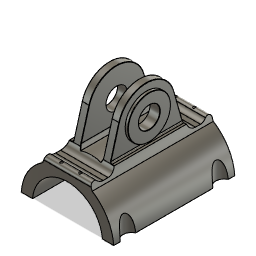
0.885.7050 - Demi-bride à chape pour tube 49 - IGTE 21485_232872 (Autodesk Fusion 360 design; units mm, degrees)
Autodesk Fusion 360 part; units mm, degrees
sketch "Sketch1" plane through (0, 0, 0) normal (0, 0, 1) x (1, 0, 0)
  line L0 (0, 0) -> (50, 0) construction
  line L1 (0, 0) -> (0, 2) construction
  line L2 (0, 0) -> (-50, 0) construction
  line L3 (0, 2) -> (50, 2) construction
  line L4 (0, 2) -> (-50, 2) construction
  arc A0 (24.5186, 2) -> (-24.5186, 2) centre (0, 0) ccw
  arc A1 (32.4384, 2) -> (-32.4384, 2) centre (0, 0) ccw
  line L5 (24.5186, 2) -> (32.4384, 2)
  line L6 (-32.4384, 2) -> (-24.5186, 2)
  line L7 (0, 50) -> (50, 50) construction
  line L8 (0, 50) -> (-50, 50) construction
  line L9 (0, 65) -> (50, 65) construction
  line L10 (0, 65) -> (-50, 65) construction
  line L11 (0, 70) -> (-50, 70) construction
  line L12 (0, 70) -> (50, 70) construction
  line L13 (0, 2) -> (0, 70) construction
  line L14 (8, 0) -> (8, 2) construction
  line L15 (8, 2) -> (8, 70) construction
  line L16 (-8, 0) -> (-8, 2) construction
  line L17 (-8, 2) -> (-8, 70) construction
  line L18 (13, 0) -> (13, 2) construction
  line L19 (-13, 0) -> (-13, 2) construction
  line L20 (-13, 2) -> (-13, 70) construction
  line L21 (15, 0) -> (15, 2) construction
  line L22 (15, 40.9995) -> (15, 65)
  line L23 (-15, 0) -> (-15, 2) construction
  line L24 (-15, 2) -> (-15, 65) construction
  arc A2 (28.931, 2) -> (-28.931, 2) centre (0, 0) ccw construction
  arc A3 (28.53, 2) -> (22.93, 17.0931) centre (0, 0) ccw
  line L25 (8, 70) -> (13, 70)
  line L26 (8, 70) -> (8, 35)
  line L27 (0, 29) -> (2, 29)
  arc A4 (2, 29) -> (8, 35) centre (2, 35) ccw
  arc A5 (-8, 35) -> (-2, 29) centre (-2, 35) ccw
  line L28 (0, 29) -> (-2, 29)
  line L29 (-8, 70) -> (-8, 35)
  line L30 (-8, 70) -> (-13, 70)
  arc A6 (15, 40.9995) -> (22.93, 17.0931) centre (55, 40.9995) ccw
  line L31 (-15, 40.9995) -> (-15, 65)
  arc A7 (-22.93, 17.0931) -> (-15, 40.9995) centre (-55, 40.9995) ccw
  arc A8 (-22.93, 17.0931) -> (-28.53, 2) centre (0, 0) ccw
  line L32 (13, 70) -> (13, 67)
  line L33 (15, 65) -> (15, 65)
  arc A9 (13, 67) -> (15, 65) centre (15, 67) ccw
  arc A10 (-15, 65) -> (-13, 67) centre (-15, 67) ccw
  line L34 (-13, 70) -> (-13, 67)
  dimension "d1" = 50
  dimension "d2" = 2
  dimension "d3" = 2
  dimension "d4" = 49.2
  dimension "d5" = 65
  dimension "d6" = 50
  dimension "d7" = 65
  dimension "d8" = 70
  dimension "d9" = 8
  dimension "d10" = 8
  dimension "d12" = 13
  dimension "d17" = 6
  dimension "d18" = 40
  dimension "d19" = 2
  constraint coincident L0.start L1.start
  constraint symmetric L0.start L1 L2.start
  constraint symmetric L0.end L1 L2.end
  constraint coincident L4 A1.end
  constraint coincident L4 A0.end
  constraint coincident L3 A0.start
  constraint coincident L3 A1.start
  constraint perpendicular L11 L13
  constraint coincident L4 A2.end
  constraint coincident L3 A2.start
  constraint coincident L3 A3.start
  constraint midpoint A2 L27.start
  constraint tangent A2 L27
  constraint perpendicular L22 L27
  constraint perpendicular L26 L27
  constraint tangent L26 A4
  constraint tangent L27 A4
  constraint symmetric L13 L15.end L17.end
  constraint symmetric L13 L25.end L20.end
  constraint symmetric L13 L27.start L28.start
  constraint symmetric L13 L26.end A5.start
  constraint symmetric L13 L27.end A5.end
  constraint symmetric L13 A4 A5
  constraint parallel L1 L21
  constraint parallel L13 L22
  constraint tangent A3 A6
  constraint tangent L22 A6
  constraint symmetric L13 A3.start A8.end
  constraint symmetric L13 A3 A8
  constraint symmetric L13 L22.start L31.start
  constraint symmetric L13 A3.end A7.start
  constraint symmetric L13 A6 A7
  constraint perpendicular L9 L32
  constraint coincident L9 L22.end
  constraint parallel L1 L18
  constraint tangent L32 A9
  constraint parallel L1 L23
  constraint parallel L13 L24
  constraint coincident L10 L24.end
  constraint symmetric L13 L22.end L24.end
  constraint symmetric L13 L32.end A10.end
  constraint symmetric L13 A9 A10
  measures "d1" distance of L0.start L0.end
  measures "d2" distance of L0.start L1.end
  measures "d4" diameter of A0
  measures "d5" diameter of A1
  measures "d6" distance of L0
  measures "d17" radius of A4
  measures "d18" radius of A6
  measures "d19" radius of A9
extrude "Extrude1" add sketch "Sketch1" along normal mid plane 85
sketch "Sketch2" plane through (0, 0, 0) normal (1, 0, 0) x (0, 0, -1)
  line L0 (42.5, 27.4786) -> (-42.5, 27.4786) construction
  line L1 (-42.5, 27.4786) -> (-42.5, 2) construction
  line L2 (-42.5, 2) -> (42.5, 2) construction
  line L3 (42.5, 2) -> (42.5, 27.4786) construction
  line L4 (42.5, 40.9995) -> (-42.5, 40.9995) construction
  line L5 (-42.5, 27.4786) -> (-42.5, 40.9995) construction
  line L6 (-42.5, 27.4786) -> (42.5, 27.4786) construction
  line L7 (42.5, 40.9995) -> (42.5, 27.4786) construction
  line L8 (42.5, 65) -> (-42.5, 65) construction
  line L9 (-42.5, 65) -> (-42.5, 40.9995) construction
  line L10 (-42.5, 40.9995) -> (42.5, 40.9995) construction
  line L11 (42.5, 40.9995) -> (42.5, 65) construction
  line L12 (42.5, 70) -> (-42.5, 70) construction
  line L13 (-42.5, 70) -> (-42.5, 67) construction
  line L14 (-42.5, 67) -> (42.5, 67) construction
  line L15 (42.5, 67) -> (42.5, 70) construction
  line L16 (42.5, 67) -> (-42.5, 67) construction
  line L17 (-42.5, 65) -> (-42.5, 67) construction
  line L18 (-42.5, 65) -> (42.5, 65) construction
  line L19 (42.5, 67) -> (42.5, 65) construction
  line L20 (0, 0) -> (0, 50) construction
  circle A0 centre (0, 50) radius 15 construction
  line L21 (0, 0) -> (70, 0) construction
  line L22 (0, 29.5) -> (70, 29.5) construction
  line L23 (42.5, 2) -> (42.5, 0) construction
  line L24 (32.5, 2) -> (32.5, 0) construction
  line L25 (32.5, 2) -> (32.5, 29.5) construction
  line L26 (38.5, 29.5) -> (38.5, 2) construction
  line L27 (26.5, 29.5) -> (26.5, 2) construction
  line L28 (25.3762, 33.5188) -> (19.2611, 55.3862)
  arc A1 (19.2611, 55.3862) -> (0, 70) centre (0, 50) ccw
  line L29 (30.673, 29.5) -> (32.5, 29.5)
  arc A2 (25.3762, 33.5188) -> (30.673, 29.5) centre (30.673, 35) ccw
  line L30 (0, 2) -> (42.5, 2)
  line L31 (42.5, 29.5) -> (42.5, 2)
  arc A3 (42.5, 29.5) -> (38.1845, 31.2187) centre (40, 29.5) ccw
  arc A4 (38.5, 27.5) -> (38.529, 27.4786) centre (40, 29.5) ccw
  line L32 (32.5, 29.5) -> (34.1905, 29.5)
  arc A5 (34.1905, 29.5) -> (38.1845, 31.2188) centre (34.1905, 35) ccw
  arc A6 (0, 70) -> (-19.2611, 55.3862) centre (0, 50) ccw
  line L33 (-25.3762, 33.5188) -> (-19.2611, 55.3862)
  arc A7 (-30.673, 29.5) -> (-25.3762, 33.5188) centre (-30.673, 35) ccw
  line L34 (-30.673, 29.5) -> (-32.5, 29.5)
  line L35 (-32.5, 29.5) -> (-34.1905, 29.5)
  arc A8 (-38.1845, 31.2188) -> (-34.1905, 29.5) centre (-34.1905, 35) ccw
  arc A9 (-38.1845, 31.2187) -> (-42.5, 29.5) centre (-40, 29.5) ccw
  line L36 (-42.5, 29.5) -> (-42.5, 2)
  line L37 (0, 2) -> (-42.5, 2)
  line L38 (42.5, 70) -> (-42.5, 70)
  line L39 (-42.5, 29.5) -> (-42.5, 70)
  line L40 (42.5, 29.5) -> (42.5, 70)
  dimension "d22" = 50
  dimension "d23" = 30
  dimension "d24" = 40
  dimension "d25" = 29.5
  dimension "d26" = 10
  dimension "d28" = 12
  dimension "d29" = 5.5
  dimension "d30" = 5
  dimension "d31" = 5.5
  constraint coincident L20.start L21.start
  constraint coincident L20.end A0.centre
  constraint concentric A0 A1
  constraint perpendicular L20 L21
  constraint coincident L2.end L3.start
  constraint coincident L21 L23.end
  constraint perpendicular L21 L23
  constraint perpendicular L22 L25
  constraint coincident L22 L25.end
  constraint coincident L22 L26.start
  constraint coincident L2 L26.end
  constraint tangent L28 A1
  constraint coincident L12 A1.end
  constraint perpendicular L25 L29
  constraint tangent L29 A2
  constraint tangent L28 A2
  constraint coincident L20 L30.start
  constraint coincident L22 L31.start
  constraint parallel L23 L31
  constraint coincident L0 A4.end
  constraint coincident L26 A4.start
  constraint concentric A3 A4
  constraint tangent L32 A5
  constraint tangent A3 A5
  constraint symmetric L20 L2.end L1.end
  constraint symmetric L20 L25.end L34.end
  constraint symmetric L20 L28.end A6.end
  constraint symmetric L20 A1.end A6.start
  constraint symmetric L20 A1 A6
  constraint symmetric L20 L29.start A7.start
  constraint symmetric L20 L28.start L33.start
  constraint symmetric L20 A2 A7
  constraint symmetric L20 L30.start L37.start
  constraint symmetric L20 L31.start A9.end
  constraint symmetric L20 A3 A9
  constraint symmetric L20 L32.end L35.end
  constraint symmetric L20 A3.end A9.start
  constraint symmetric L20 A5 A8
  constraint coincident L12.start L15.end
  constraint coincident L12.end L13.start
  constraint tangent A9 L39
  measures "d22" distance of L20.start L20.end
  measures "d23" diameter of A0
  measures "d24" diameter of A1
  measures "d29" radius of A2
  measures "d30" diameter of A3
  measures "d31" radius of A5
extrude "Extrude2" cut sketch "Sketch2" along normal through all and the other way through all contours L28 A1 L29 A2 A3 L32 A5 L38 L40 | A6 L33 A7 L34 L35 A8 A9 L38 L39
sketch "Sketch3" plane through (0, 0, 0) normal (1, 0, 0) x (0, 0, -1)
  spline S0 degree 3 poles (-42.5, 29.5) (-42.5, 29.8124) (-42.4379, 30.1478) (-42.1803, 30.7685) (-41.9847, 31.0537) (-41.5367, 31.4959) (-41.2582, 31.6855) (-40.6464, 31.9375) (-40.3131, 32) (-40, 32) (-39.6869, 32) (-39.3536, 31.9375) (-38.7418, 31.6855) (-38.4633, 31.4959) (-38.2239, 31.2596) (-38.2041, 31.2394) (-38.1845, 31.2187) knots -0.383515 -0.383515 -0.383515 -0.383515 -0.285675 -0.285675 -0.187835 -0.187835 -0.093917 -0.093917 0 0 0 0.093917 0.093917 0.187835 0.187835 0.196405 0.196405 0.196405 0.196405
  line L0 (-38.1845, 31.2188) -> (-42.5, 29.5)
  spline S1 degree 3 poles (38.1845, 31.2187) (38.2041, 31.2394) (38.2239, 31.2596) (38.4633, 31.4959) (38.7418, 31.6855) (39.3536, 31.9375) (39.6869, 32) (40, 32) (40.3131, 32) (40.6464, 31.9375) (41.2582, 31.6855) (41.5367, 31.4959) (41.9847, 31.0537) (42.1803, 30.7685) (42.4379, 30.1478) (42.5, 29.8124) (42.5, 29.5) knots -0.196405 -0.196405 -0.196405 -0.196405 -0.187835 -0.187835 -0.093917 -0.093917 0 0 0 0.093917 0.093917 0.187835 0.187835 0.285675 0.285675 0.383515 0.383515 0.383515 0.383515
  line L1 (42.5, 29.5) -> (38.1845, 31.2187)
  constraint coincident S0.start L0.end
  constraint coincident S1.end L1.start
  constraint coincident S1.start L1.end
extrude "Extrude3" add sketch "Sketch3" along normal mid plane 19
sketch "Sketch4" plane through (0, 0, 0) normal (1, 0, 0) x (0, 0, -1)
  line L0 (0, 0) -> (0, 50)
  circle A0 centre (0, 50) radius 7.5
  dimension "d36" = 50
  dimension "d37" = 15
  constraint coincident L0.start origin
  constraint coincident L0.end A0.centre
  measures "d36" distance of L0.start L0.end
  measures "d37" diameter of A0
extrude "Extrude4" cut sketch "Sketch4" along normal through all and the other way through all
sketch "Sketch5" plane through (0, 0, 0) normal (0, 1, 0) x (1, 0, 0)
  line L0 (-32.4384, 42.5) -> (-32.4384, -42.5) construction
  line L1 (-32.4384, -42.5) -> (-24.5186, -42.5) construction
  line L2 (24.5186, -42.5) -> (32.4384, -42.5) construction
  line L3 (24.5186, -42.5) -> (-24.5186, -42.5) construction
  line L4 (32.4384, 42.5) -> (32.4384, -42.5) construction
  line L5 (-24.5186, 42.5) -> (-32.4384, 42.5) construction
  line L6 (-24.5186, 42.5) -> (24.5186, 42.5) construction
  line L7 (32.4384, 42.5) -> (24.5186, 42.5) construction
  line L8 (-24.5186, 32.5) -> (24.5186, 32.5) construction
  line L9 (24.5186, -32.5) -> (-24.5186, -32.5) construction
  line L10 (24.5186, 32.5) -> (32.4384, 32.5) construction
  line L11 (24.5186, -32.5) -> (32.4384, -32.5) construction
  line L12 (-24.5186, -32.5) -> (-32.4384, -32.5) construction
  line L13 (-24.5186, 32.5) -> (-32.4384, 32.5) construction
  line L14 (0, -42.5) -> (0, 42.5) construction
  line L15 (0, -32.5) -> (-35, -32.5) construction
  circle A0 centre (-35, -32.5) radius 6
  line L16 (-32.4384, 0) -> (32.4384, 0) construction
  circle A1 centre (-35, 32.5) radius 6
  circle A2 centre (35, -32.5) radius 6
  circle A3 centre (35, 32.5) radius 6
  dimension "d40" = 10
  dimension "d41" = 10
  dimension "d42" = 35
  dimension "d43" = 12
  constraint horizontal L10
  constraint perpendicular L4 L11
  constraint perpendicular L0 L12
  constraint perpendicular L0 L13
  constraint coincident L0 L13.end
  constraint coincident L0 L12.end
  constraint coincident L4 L11.end
  constraint coincident L4 L10.end
  constraint midpoint L3 L14.start
  constraint midpoint L6 L14.end
  constraint midpoint L9 L15.start
  constraint coincident L15.end A0.centre
  constraint midpoint L0 L16.start
  constraint midpoint L4 L16.end
  constraint symmetric A0 L16 A1
  constraint symmetric L14 A0 A2
  constraint symmetric L14 A1 A3
  measures "d42" distance of L15.start L15.end
  measures "d43" diameter of A0
extrude "Extrude5" cut sketch "Sketch5" along normal blind 65
sketch "Sketch6" plane through (15, 0, 0) normal (1, 0, 0) x (0, 0, -1)
  circle A0 centre (0, 50) radius 7.5 construction
  line L0 (23.2842, 40.9995) -> (19.2611, 55.3862) construction
  arc A1 (19.2611, 55.3862) -> (13.2288, 65) centre (0, 50) ccw construction
  line L1 (13.2288, 65) -> (-13.2288, 65) construction
  arc A2 (-13.2288, 65) -> (-19.2611, 55.3862) centre (0, 50) ccw
  line L2 (-19.2611, 55.3862) -> (-23.2842, 40.9995)
  line L3 (-23.2842, 40.9995) -> (23.2842, 40.9995) construction
  circle A3 centre (0, 50) radius 7.5 construction
  line L4 (-24.962, 35) -> (-19.2611, 55.3862)
  arc A4 (19.2611, 55.3862) -> (-19.2611, 55.3862) centre (0, 50) ccw
  line L5 (19.2611, 55.3862) -> (24.962, 35)
  line L6 (24.962, 35) -> (-24.962, 35)
  line L7 (13.2288, 65) -> (-13.2288, 65) construction
  line L8 (10.5357, 67) -> (-10.5357, 67) construction
  line L9 (23.2842, 40.9995) -> (-23.2842, 40.9995) construction
  line L10 (42.5, 27.4786) -> (-42.5, 27.4786) construction
  circle A5 centre (0, 50) radius 15
  dimension "d46" = 30
  constraint concentric A0 A5
  measures "d46" diameter of A5
extrude "Extrude6" cut sketch "Sketch6" against normal blind 2
sketch "Sketch7" plane through (13, 0, 0) normal (1, 0, 0) x (0, 0, -1)
  arc A0 (19.2611, 55.3862) -> (-19.2611, 55.3862) centre (0, 50) ccw
  line L0 (-19.2611, 55.3862) -> (-24.962, 35)
  line L1 (-24.962, 35) -> (0.001, 35)
  circle A1 centre (0, 50) radius 15
  line L2 (0.001, 35) -> (24.962, 35)
  line L3 (24.962, 35) -> (19.2611, 55.3862)
  line L4 (0.001, 35) -> (-24.962, 35)
  line L5 (-24.962, 35) -> (-19.2611, 55.3862)
  arc A2 (19.2611, 55.3862) -> (-19.2611, 55.3862) centre (0, 50) ccw
  line L6 (19.2611, 55.3862) -> (24.962, 35)
  line L7 (24.962, 35) -> (23.2842, 40.9995)
  line L8 (25.3762, 33.5188) -> (23.2842, 40.9995)
  line L9 (25.3762, 33.5188) -> (24.962, 35)
  line L10 (24.962, 35) -> (19.2611, 55.3862)
  line L11 (19.2611, 55.3862) -> (24.962, 35)
  line L12 (-23.2842, 40.9995) -> (-24.962, 35)
  line L13 (-24.962, 35) -> (-19.2611, 55.3862)
  line L14 (-19.2611, 55.3862) -> (-24.962, 35)
  line L15 (-24.962, 35) -> (-25.3762, 33.5188)
  line L16 (-23.2842, 40.9995) -> (-25.3762, 33.5188)
  line L17 (25.3762, 33.5188) -> (-25.3762, 33.5188)
  constraint coincident L8.start L9.start
  constraint coincident L15.end L16.end
extrude "Extrude7" cut sketch "Sketch7" along normal blind 8 contours A0 L0 L1 L2 L3 L4 L5 A2 L6 L7 L8 L10 L11 L12 L13 L14 L16
sketch "Sketch8" plane through (13, 0, 0) normal (1, 0, 0) x (0, 0, -1)
  arc A0 (19.2611, 55.3862) -> (-19.2611, 55.3862) centre (0, 50) ccw
  line L0 (-19.2611, 55.3862) -> (-24.962, 35)
  line L1 (-24.962, 35) -> (0.001, 35)
  circle A1 centre (0, 50) radius 15
  line L2 (0.001, 35) -> (24.962, 35)
  line L3 (24.962, 35) -> (19.2611, 55.3862)
  line L4 (19.2611, 55.3862) -> (24.962, 35)
  line L5 (25.3762, 33.5188) -> (24.962, 35)
  line L6 (-24.962, 35) -> (-25.3762, 33.5188)
  line L7 (-24.962, 35) -> (-19.2611, 55.3862)
  arc A2 (19.2611, 55.3862) -> (-19.2611, 55.3862) centre (0, 50) ccw
  line L8 (25.3762, 33.5188) -> (-25.3762, 33.5188)
  constraint coincident L5.start L8.start
  constraint coincident L6.end L8.end
extrude "Extrude8" cut sketch "Sketch8" along normal blind 17 contours L1 L2 L5 L6 L8
sketch "Sketch12" plane through (-13, 0, 0) normal (-1, 0, 0) x (0, 0, 1)
  arc A0 (10.5357, 67) -> (-10.5357, 67) centre (0, 50) ccw
  line L0 (-10.5357, 67) -> (10.5357, 67)
  circle A1 centre (0, 50) radius 15
  line L1 (19.2611, 55.3862) -> (25.3762, 33.5188)
  line L2 (25.3762, 33.5188) -> (-25.3762, 33.5188)
  line L3 (-25.3762, 33.5188) -> (-19.2611, 55.3862)
  arc A2 (19.2611, 55.3862) -> (-19.2611, 55.3862) centre (0, 50) ccw
extrude "Extrude11" cut sketch "Sketch12" along normal blind 12
sketch "Sketch13" plane through (0, 0, 0) normal (0, 0, 1) x (1, 0, 0)
  line L0 (15, 40.9995) -> (15, 65) construction
  spline S0 degree 3 poles (15, 40.9995) (15, 40.4363) (15.0119, 39.9103) (15.0836, 38.0858) (15.2006, 36.9234) (15.3419, 35.7661) (15.383, 35.4742) (15.4383, 35.0911) (15.4468, 35.0364) (15.4525, 35) (15.4525, 35) (15.4525, 35) knots 3.304882 3.304882 3.304882 3.304882 3.508507 3.508507 4.076666 4.076666 4.360745 4.360745 4.644824 4.644824 4.644928 4.644928 4.644928 4.644928 construction
  line L1 (15, 40.9995) -> (15, 65) construction
  spline S1 degree 3 poles (15.4525, 35) (15.4525, 35.0001) (15.4383, 35.0912) (15.383, 35.4742) (15.3419, 35.7661) (15.2006, 36.9234) (15.0836, 38.0858) (15.0119, 39.9103) (15, 40.4363) (15, 40.9995) knots 4.644928 4.644928 4.644928 4.644928 4.928904 4.928904 5.212983 5.212983 5.781142 5.781142 5.984766 5.984766 5.984766 5.984766 construction
  line L2 (13, 35) -> (13, 65) construction
  line L3 (15, 65) -> (18, 65)
  line L4 (18, 65) -> (18, 34)
  line L5 (18, 34) -> (15, 34)
  line L6 (15, 34) -> (15, 65)
  line L7 (16.6886, 29.5) -> (-16.6886, 29.5)
  line L8 (-16.2142, 31.2187) -> (16.2142, 31.2187)
  line L9 (0, 29.5) -> (0, 63) construction
  line L10 (-18, 65) -> (-18, 34)
  line L11 (-15, 65) -> (-18, 65)
  line L12 (-15, 34) -> (-15, 65)
  line L13 (-18, 34) -> (-15, 34)
  constraint horizontal L3
  constraint vertical L4
  constraint horizontal L5
  constraint vertical L6
  constraint coincident L0.end L1.end
  constraint midpoint L7 L9.start
  constraint perpendicular L8 L9
  constraint symmetric L3.end L9 L10.start
  constraint symmetric L4.end L9 L10.end
  constraint symmetric L0.end L9 L11.start
  constraint symmetric L5.end L9 L12.start
extrude "Extrude12" cut sketch "Sketch13" along normal through all and the other way through all
fillet "Fillet2" radius 1 2 edges at (13, 33.5188, 0) (-13, 33.5188, 0)
fillet "Fillet3" radius 0.2 32 edges at (15, 44.5758, 13.9849) (14.8529, 33.5188, -25.3762) (13.2929, 33.8117, -25.2943) (13, 44.9525, -22.1788) (13, 70, 0) (13, 44.9525, 22.1788) (13.2929, 33.8117, 25.2943) (14.8529, 33.5188, 25.3762) (15, 52.7121, 6.9925) (7.4843, 32.5665, 25.7407) (7.9534, 34.2536, 25.1707) (8, 45.1931, 22.1115) (8, 70, 0) (8, 45.1931, -22.1115) (7.9534, 34.2536, -25.1707) (7.4843, 32.5665, -25.7407) (-7.4843, 32.5665, -25.7407) (-7.9534, 34.2536, -25.1707) (-8, 45.1931, -22.1115) (-8, 70, 0) (-8, 45.1931, 22.1115) (-7.9534, 34.2536, 25.1707) (-7.4843, 32.5665, 25.7407) (-14.8529, 33.5188, -25.3762) (-13.2929, 33.8117, -25.2943) (-13, 44.9525, -22.1788) (-13, 70, 0) (-13, 44.9525, 22.1788) (-13.2929, 33.8117, 25.2943) (-14.8529, 33.5188, 25.3762) (-15, 55.4242, -13.9849) (-15, 47.2879, 6.9925)
equation "d4 = ( 24.6 * 2 ) * 1 mm"
equation "d5 = ( 32.5 * 2 ) * 1 mm"
